Autodesk Fusion 360 part; units mm, degrees
(part 4 of 4)
sketch "Esquisse2 (5)" plane through (0, 0, 5) normal (0, 0, 1) x (-1, 0, 0) in component "Wood_Side_Left"
  line L0 (57.7939, -16.8522) -> (57.7939, 53.1478)
  line L1 (57.7939, 53.1478) -> (-242.2061, 53.1478)
  line L2 (-242.2061, 53.1478) -> (-242.2061, -16.8522)
  line L3 (-242.2061, -16.8522) -> (57.7939, -16.8522)
  line L4 (-117.7061, 31.1478) -> (-66.7061, 31.1478) construction
  line L5 (-66.7061, 31.1478) -> (-66.7061, 5.1478) construction
  line L6 (-66.7061, 5.1478) -> (-117.7061, 5.1478) construction
  line L7 (-117.7061, 5.1478) -> (-117.7061, 31.1478) construction
  line L8 (-66.4061, 4.8478) -> (-118.0061, 4.8478)
  line L9 (-118.0061, 4.8478) -> (-118.0061, 31.4478)
  line L10 (-118.0061, 31.4478) -> (-66.4061, 31.4478)
  line L11 (-66.4061, 31.4478) -> (-66.4061, 4.8478)
  circle A0 centre (-63.4061, 18.1478) radius 1.65
  circle A1 centre (-121.0061, 18.1478) radius 1.65
  circle A2 centre (-231.9061, 3.1478) radius 1.65
  circle A3 centre (-164.4061, -6.8522) radius 1.65
  circle A4 centre (-19.4061, -6.8522) radius 1.65
  circle A5 centre (48.0939, 3.1478) radius 1.65
  dimension "d451" = 3.3
  dimension "d452" = 3.3
  constraint horizontal L4
  constraint vertical L5
  constraint horizontal L6
  constraint vertical L7
  measures "d451" diameter of A0
  measures "d452" diameter of A1
sketch "Esquisse2 (6)" plane through (0, 0, 5) normal (0, 0, 1) x (-1, 0, 0) in component "Wood_Front"
  line L0 (-110, -30) -> (140, -30)
  line L1 (140, -30) -> (140, 40)
  line L2 (140, 40) -> (-110, 40)
  line L3 (-110, 40) -> (-110, -30)
  line L4 (-10.5, 18) -> (40.5, 18) construction
  line L5 (40.5, 18) -> (40.5, -8) construction
  line L6 (40.5, -8) -> (-10.5, -8) construction
  line L7 (-10.5, -8) -> (-10.5, 18) construction
  line L8 (40.8, -8.3) -> (-10.8, -8.3)
  line L9 (-10.8, -8.3) -> (-10.8, 18.3)
  line L10 (-10.8, 18.3) -> (40.8, 18.3)
  line L11 (40.8, 18.3) -> (40.8, -8.3)
  circle A0 centre (43.8, 5) radius 1.65
  circle A1 centre (-13.8, 5) radius 1.65
  circle A2 centre (-100.9, -10) radius 1.65
  circle A3 centre (-45.75, -20) radius 1.65
  circle A4 centre (74.55, -20) radius 1.65
  circle A5 centre (129.7, -10) radius 1.65
  dimension "d449" = 3.3
  dimension "d450" = 3.3
  constraint horizontal L4
  constraint vertical L5
  constraint horizontal L6
  constraint vertical L7
  measures "d449" diameter of A0
  measures "d450" diameter of A1
sketch "Esquisse2 (7)" plane through (0, 0, 0) normal (0, 0, 1) x (1, 0, 0) in component "Wood_Side_Right"
  circle A0 centre (63.4061, -18.1478) radius 1.65
  circle A1 centre (121.0061, -18.1478) radius 1.65
  line L0 (66.7061, -31.1478) -> (117.7061, -31.1478)
  line L1 (117.7061, -31.1478) -> (117.7061, -5.1478)
  line L2 (117.7061, -5.1478) -> (66.7061, -5.1478)
  line L3 (66.7061, -5.1478) -> (66.7061, -31.1478)
  line L4 (117.4061, -5.4478) -> (67.0061, -5.4478) construction
  line L5 (67.0061, -5.4478) -> (67.0061, -30.8478) construction
  line L6 (67.0061, -30.8478) -> (117.4061, -30.8478) construction
  line L7 (117.4061, -30.8478) -> (117.4061, -5.4478) construction
  circle A2 centre (-47.4939, -3.1478) radius 1.65
  circle A3 centre (20.0061, 6.8522) radius 1.65
  circle A4 centre (165.0061, 6.8522) radius 1.65
  circle A5 centre (232.5061, -3.1478) radius 1.65
  constraint horizontal L0
  constraint vertical L1
  constraint horizontal L2
  constraint vertical L3
component "Wood_Bottom" placed x (-1, 0, 0) y (0, -1, 0) z (0, 0, 1) at (0, 0, -0.15)
component "Right_Bottom_Holder" placed x (-1, 0, 0) y (0, -1, 0) z (0, 0, 1) at (-120.3, 0, -47.2937)
component "Left_Bottom_Holder" placed x (1, 0, 0) y (0, 1, 0) z (0, 0, 1) at (120.3, 0, -47.2937)
component "Right_Top_Holder" placed x (-1, 0, 0) y (0, 1, 0) z (0, 0, -1) at (-120.3, 0, 132.2937)
component "Left_Top_Holder" placed x (1, 0, 0) y (0, -1, 0) z (0, 0, -1) at (120.3, 0, 132.2937)
component "Wood_Top" placed x (-1, 0, 0) y (0, -1, 0) z (0, 0, 1) at (0, 0.3, 80.15)
component "Wood_Side_Left" placed x (0, -1, 0) y (0, 0, -1) z (1, 0, 0) at (127.8, 91.9061, 24.3522)
component "Wood_Side_Right" placed x (0, -1, 0) y (0, 0, -1) z (1, 0, 0) at (-132.8, 92.5061, 24.3522)
component "Wood_Front" placed x (-1, 0, 0) y (0, 0, -1) z (0, -1, 0) at (-14.4, -152.5, 37.5)
component "Wood_Back" placed x (-1, 0, 0) y (0, 0, -1) z (0, -1, 0) at (-15.6, 157.5, 37.5)
component "Holding_Plate" placed x (-1, 0, 0) y (0, 0, -1) z (0, -1, 0) at (-114.5991, -161.7, 63.768)
component "Holding_Plate" placed x (-1, 0, 0) y (0, 0, -1) z (0, -1, 0) at (143.8009, -161.7, 63.768)
component "Holding_Plate" placed x (1, 0, 0) y (0, 0, -1) z (0, 1, 0) at (114.5991, 161.7, 63.768)
component "Holding_Plate" placed x (1, 0, 0) y (0, 0, -1) z (0, 1, 0) at (-143.8009, 161.7, 63.768)
equation "wood_thickness = 5 mm + insert_slot_extra_tolerance" comment "Wood thickness with extra tolerance (needs to be reduced to 5mm for panels)"
equation "bottom_panel_length = 300 mm" comment "Length of wood base plate"
equation "bottom_panel_width = 250 mm" comment "Width of wood base plate"
equation "d4 = bottom_panel_width"
equation "d5 = bottom_panel_length"
equation "d6 = wood_thickness - insert_slot_extra_tolerance"
equation "frame_height = wood_thickness + 15 mm" comment "Main holding bloc height"
equation "frame_arm_width = 20 mm" comment "Main holding bloc width"
equation "frame_length = bottom_panel_length + 2 * frame_arm_width - 2 * inset" comment "Main holding bloc length"
equation "d11 = frame_length"
equation "d12 = frame_height"
equation "d13 = frame_arm_width"
equation "tolerance = 0.3 mm"
equation "d16 = wood_thickness + tolerance"
equation "d17 = bottom_panel_length + 2 * tolerance"
equation "side_sled_width = 10 mm" comment "Width of screw connecting part on the side"
equation "inset = 5 mm" comment "Removed depth of main side block"
equation "d20 = -inset"
equation "d23 = side_sled_width"
equation "d28 = tolerance"
equation "connecting_pin_diameter = 5 mm" comment "Connecting pin diameter"
equation "connecting_pin_length = 10 mm" comment "Connecting pin length"
equation "front_rear_sled_length = 140 mm" comment "Length of part that will connect to the side of the panel using screws"
equation "sled_lip_thickness = 2.5 mm" comment "Thickness of one part of the screw connecting element"
equation "front_rear_sled_width = 15 mm" comment "Width of screw connecting part for front and rear"
equation "side_panel_height = 70 mm"
equation "d109 = frame_arm_width"
equation "d110 = frame_height"
equation "d111 = frame_arm_width"
equation "d112 = frame_height"
equation "d115 = bottom_panel_width / 2 - inset + tolerance"
equation "d117 = connecting_pin_diameter + tolerance"
equation "d118 = wood_thickness + tolerance"
equation "d119 = inset + tolerance"
equation "d120 = -tolerance - connecting_pin_length"
equation "d122 = -frame_arm_width + inset + tolerance"
equation "d124 = sled_lip_thickness"
equation "d125 = front_rear_sled_length / 4"
equation "d126 = side_sled_width"
equation "d128 = sled_lip_thickness"
equation "d129 = front_rear_sled_length / 4"
equation "d130 = side_sled_width"
equation "d134 = connecting_pin_diameter + tolerance"
equation "d135 = inset + tolerance"
equation "d136 = wood_thickness + tolerance"
equation "d137 = -connecting_pin_length - tolerance"
equation "d139 = -frame_arm_width + inset + tolerance"
equation "d141 = sled_lip_thickness"
equation "d142 = front_rear_sled_length / 4"
equation "d143 = side_sled_width"
equation "d145 = wood_thickness + tolerance"
equation "d146 = bottom_panel_length + 2 * tolerance"
equation "d149 = sled_lip_thickness"
equation "d150 = front_rear_sled_length / 4"
equation "d151 = -inset - tolerance"
equation "d153 = side_panel_height / 2 - inset"
equation "d158 = connecting_pin_diameter"
equation "d159 = connecting_pin_length"
equation "d161 = connecting_pin_diameter + tolerance"
equation "d162 = -connecting_pin_length - tolerance"
equation "d164 = connecting_pin_diameter"
equation "d165 = connecting_pin_length"
equation "d171 = sled_lip_thickness"
equation "d172 = side_panel_height / 4"
equation "d173 = side_sled_width"
equation "d175 = sled_lip_thickness"
equation "d176 = side_panel_height / 4"
equation "d177 = side_sled_width"
equation "d11_1 = frame_length"
equation "d12_1 = frame_height"
equation "d13_1 = frame_arm_width"
equation "d16_1 = wood_thickness + tolerance"
equation "d17_1 = bottom_panel_length + 2 * tolerance"
equation "d20_1 = -inset"
equation "d23_1 = side_sled_width"
equation "d109_1 = frame_arm_width"
equation "d110_1 = frame_height"
equation "d111_1 = frame_arm_width"
equation "d112_1 = frame_height"
equation "d115_1 = bottom_panel_width / 2 - inset + tolerance"
equation "d117_1 = connecting_pin_diameter"
equation "d118_1 = wood_thickness + tolerance"
equation "d119_1 = inset + tolerance"
equation "d120_1 = connecting_pin_length"
equation "d122_1 = -frame_arm_width + inset + tolerance"
equation "d124_1 = sled_lip_thickness"
equation "d125_1 = front_rear_sled_length / 4"
equation "d126_1 = side_sled_width"
equation "d128_1 = sled_lip_thickness"
equation "d129_1 = front_rear_sled_length / 4"
equation "d130_1 = side_sled_width"
equation "d134_1 = connecting_pin_diameter"
equation "d135_1 = inset + tolerance"
equation "d136_1 = wood_thickness + tolerance"
equation "d137_1 = connecting_pin_length"
equation "d139_1 = -frame_arm_width + inset + tolerance"
equation "d141_1 = sled_lip_thickness"
equation "d142_1 = front_rear_sled_length / 4"
equation "d143_1 = side_sled_width"
equation "d145_1 = wood_thickness + tolerance"
equation "d146_1 = bottom_panel_length + 2 * tolerance"
equation "d149_1 = sled_lip_thickness"
equation "d150_1 = front_rear_sled_length / 4"
equation "d151_1 = -inset - tolerance"
equation "d153_1 = side_panel_height / 2 - inset"
equation "d155_1 = connecting_pin_diameter"
equation "d156_1 = connecting_pin_length"
equation "d161_1 = connecting_pin_diameter + tolerance"
equation "d162_1 = -connecting_pin_length - tolerance"
equation "d164_1 = connecting_pin_diameter"
equation "d165_1 = connecting_pin_length"
equation "d171_1 = sled_lip_thickness"
equation "d172_1 = side_panel_height / 4"
equation "d173_1 = side_sled_width"
equation "d175_1 = sled_lip_thickness"
equation "d176_1 = side_panel_height / 4"
equation "d177_1 = side_sled_width"
equation "d11_2 = frame_length"
equation "d12_2 = frame_height"
equation "d13_2 = frame_arm_width"
equation "d16_2 = wood_thickness + tolerance"
equation "d17_2 = bottom_panel_length + 2 * tolerance"
equation "d20_2 = -inset"
equation "d23_2 = side_sled_width"
equation "d109_2 = frame_arm_width"
equation "d110_2 = frame_height"
equation "d111_2 = frame_arm_width"
equation "d112_2 = frame_height"
equation "d115_2 = bottom_panel_width / 2 - inset + tolerance"
equation "d117_2 = connecting_pin_diameter + tolerance"
equation "d118_2 = wood_thickness + tolerance"
equation "d119_2 = inset + tolerance"
equation "d120_2 = -tolerance - connecting_pin_length"
equation "d122_2 = -frame_arm_width + inset + tolerance"
equation "d124_2 = sled_lip_thickness"
equation "d125_2 = front_rear_sled_length / 4"
equation "d126_2 = side_sled_width"
equation "d134_2 = connecting_pin_diameter + tolerance"
equation "d135_2 = inset + tolerance"
equation "d136_2 = wood_thickness + tolerance"
equation "d137_2 = -connecting_pin_length - tolerance"
equation "d139_2 = -frame_arm_width + inset + tolerance"
equation "d141_2 = sled_lip_thickness"
equation "d142_2 = front_rear_sled_length / 4"
equation "d143_2 = side_sled_width"
equation "d145_2 = wood_thickness + tolerance"
equation "d146_2 = bottom_panel_length + 2 * tolerance"
equation "d151_2 = -inset - tolerance"
equation "d153_2 = side_panel_height / 2 - inset"
equation "d156_2 = -connecting_pin_length - tolerance"
equation "d161_2 = connecting_pin_diameter + tolerance"
equation "d162_2 = -connecting_pin_length - tolerance"
equation "d164_2 = connecting_pin_diameter"
equation "d165_2 = connecting_pin_length"
equation "d11_1_1 = frame_length"
equation "d12_1_1 = frame_height"
equation "d13_1_1 = frame_arm_width"
equation "d16_1_1 = wood_thickness + tolerance"
equation "d17_1_1 = bottom_panel_length + 2 * tolerance"
equation "d20_1_1 = -inset"
equation "d109_1_1 = frame_arm_width"
equation "d110_1_1 = frame_height"
equation "d111_1_1 = frame_arm_width"
equation "d112_1_1 = frame_height"
equation "d115_1_1 = bottom_panel_width / 2 - inset + tolerance"
equation "d117_1_1 = connecting_pin_diameter"
equation "d118_1_1 = wood_thickness + tolerance"
equation "d119_1_1 = inset + tolerance"
equation "d120_1_1 = connecting_pin_length"
equation "d122_1_1 = -frame_arm_width + inset + tolerance"
equation "d134_1_1 = connecting_pin_diameter"
equation "d135_1_1 = inset + tolerance"
equation "d136_1_1 = wood_thickness + tolerance"
equation "d137_1_1 = connecting_pin_length"
equation "d139_1_1 = -frame_arm_width + inset + tolerance"
equation "d145_1_1 = wood_thickness + tolerance"
equation "d146_1_1 = bottom_panel_length + 2 * tolerance"
equation "d151_1_1 = -inset - tolerance"
equation "d153_1_1 = side_panel_height / 2 - inset"
equation "d155_1_1 = connecting_pin_diameter + tolerance"
equation "d156_1_1 = -connecting_pin_length - tolerance"
equation "d161_1_1 = connecting_pin_diameter + tolerance"
equation "d162_1_1 = -connecting_pin_length - tolerance"
equation "d164_1_1 = connecting_pin_diameter"
equation "d165_1_1 = connecting_pin_length"
equation "d4_1 = bottom_panel_width"
equation "d5_1 = bottom_panel_length"
equation "d6_1 = wood_thickness - insert_slot_extra_tolerance"
equation "d195 = bottom_panel_length"
equation "d196 = side_panel_height"
equation "d197 = wood_thickness - insert_slot_extra_tolerance"
equation "d195_1 = bottom_panel_length"
equation "d196_1 = side_panel_height"
equation "d197_1 = wood_thickness - insert_slot_extra_tolerance"
equation "d207 = bottom_panel_width"
equation "d208 = side_panel_height"
equation "d209 = wood_thickness - insert_slot_extra_tolerance"
equation "d207_1 = bottom_panel_width"
equation "d208_1 = side_panel_height"
equation "d209_1 = wood_thickness - insert_slot_extra_tolerance"
equation "d230 = sled_lip_thickness"
equation "d231 = front_rear_sled_length / 4"
equation "d232 = sled_lip_thickness"
equation "d233 = front_rear_sled_length / 4"
equation "d234 = sled_lip_thickness"
equation "d235 = front_rear_sled_length / 4"
equation "d236 = sled_lip_thickness"
equation "d237 = front_rear_sled_length / 4"
equation "d238 = sled_lip_thickness"
equation "d239 = front_rear_sled_length / 4"
equation "screw_hole_diameter = 3.3 mm" comment "Hole diameter for good fit for M3 screws"
equation "d247 = screw_hole_diameter"
equation "d248 = screw_hole_diameter"
equation "d249 = screw_hole_diameter"
equation "d250 = screw_hole_diameter"
equation "d253 = screw_hole_diameter"
equation "d254 = screw_hole_diameter"
equation "d255 = screw_hole_diameter"
equation "d256 = screw_hole_diameter"
equation "d260 = screw_hole_diameter"
equation "d263 = screw_hole_diameter"
equation "d264 = screw_hole_diameter"
equation "d265 = screw_hole_diameter"
equation "d266 = screw_hole_diameter"
equation "d270 = screw_hole_diameter"
equation "d271 = screw_hole_diameter"
equation "d272 = screw_hole_diameter"
equation "d273 = screw_hole_diameter"
equation "d278 = screw_hole_diameter"
equation "d285 = screw_hole_diameter"
equation "d286 = screw_hole_diameter"
equation "d287 = screw_hole_diameter"
equation "d288 = screw_hole_diameter"
equation "d323 = sled_lip_thickness"
equation "d324 = side_panel_height / 4"
equation "d325 = sled_lip_thickness"
equation "d326 = side_panel_height / 4"
equation "d327 = side_sled_width"
equation "d329 = screw_hole_diameter"
equation "d330 = sled_lip_thickness"
equation "d331 = side_panel_height / 4"
equation "d332 = sled_lip_thickness"
equation "d333 = side_panel_height / 4"
equation "d334 = side_sled_width"
equation "d336 = screw_hole_diameter"
equation "inserts_hole_diameter = 5.60 mm" comment "Hole diameter to fit the M3 inserts"
equation "inserts_hole_depth = 4.2 mm" comment "Hole depth for M3 inserts"
equation "holding_plate_thickness = 3 mm" comment "Thickness of plate that will connect the frame parts"
equation "holding_plate_length = 30 mm"
equation "d343 = holding_plate_length / 2 + tolerance"
equation "d344 = inserts_hole_diameter"
equation "holding_plate_width = 10 mm" comment "Width of the holding plate"
equation "d346 = holding_plate_width + tolerance"
equation "d347 = -holding_plate_thickness - tolerance"
equation "d349 = -inserts_hole_depth"
equation "connecting_pin_side_distance = 10 mm" comment "Distance of pin to side where there is a connecting plate"
equation "d354 = connecting_pin_diameter"
equation "d355 = -holding_plate_thickness - tolerance"
equation "d358 = -inserts_hole_depth"
equation "d360 = connecting_pin_diameter + tolerance"
equation "d361 = connecting_pin_diameter + tolerance"
equation "d362 = holding_plate_width + tolerance"
equation "d363 = holding_plate_length / 2 + tolerance"
equation "d364 = inserts_hole_diameter"
equation "d365 = -holding_plate_thickness - tolerance"
equation "d368 = -inserts_hole_depth"
equation "d370 = -holding_plate_thickness - tolerance"
equation "d373 = -inserts_hole_depth"
equation "d375 = connecting_pin_diameter"
equation "d376 = holding_plate_length / 2 + tolerance"
equation "d377 = holding_plate_width + tolerance"
equation "d378 = inserts_hole_diameter"
equation "d379 = -holding_plate_thickness - tolerance"
equation "d382 = -inserts_hole_depth"
equation "d384 = -holding_plate_thickness - tolerance"
equation "d390 = -inserts_hole_depth"
equation "d392 = connecting_pin_diameter + tolerance"
equation "d393 = holding_plate_length / 2 + tolerance"
equation "d394 = holding_plate_width + tolerance"
equation "d395 = inserts_hole_diameter"
equation "d396 = -holding_plate_thickness - tolerance"
equation "d399 = -inserts_hole_depth"
equation "d401 = -holding_plate_thickness - tolerance"
equation "d404 = -inserts_hole_depth"
equation "d406 = holding_plate_width"
equation "d407 = holding_plate_length"
equation "d408 = holding_plate_length / 4 + tolerance"
equation "d409 = holding_plate_thickness"
equation "M3_screw_head_diameter = 6 mm"
equation "M3_screw_head_thickness = 2.40 mm"
equation "d413 = M3_screw_head_diameter"
equation "d414 = screw_hole_diameter"
equation "d416 = -M3_screw_head_thickness"
equation "d438 = -tolerance"
equation "d443 = -tolerance"
equation "d448 = -tolerance"
equation "insert_slot_extra_tolerance = 0.30 mm" comment "Additional tolerance for part where wood panel is inserted"
named bodies: "Wood_Bottom", "Side_Holder", "Side_Holder (1)", "Wood_Top", "Wood_Side_Left", "Wood_Side_Right", "Wood_Front", "Wood_Back", "Holding_Plate"
